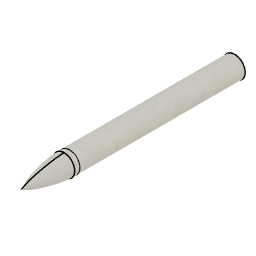
Rocket- Main Body with nosecone_ (Autodesk Fusion 360 design; units mm, degrees)
Autodesk Fusion 360 part; units mm, degrees
sketch "Rocket Nose" plane through (0, 0, 0) normal (1, 0, 0) x (0, 1, 0)
  spline S0 degree 5 poles (152.4, 0) (151.241, 0.6822) (148.9185, 2.0223) (145.4215, 3.9595) (140.7321, 6.3961) (134.8257, 9.1975) (128.8755, 11.7569) (122.883, 14.0821) (116.8517, 16.1887) (110.7874, 18.1036) (104.6973, 19.8612) (98.589, 21.4976) (92.4695, 23.0466) (86.3443, 24.5345) (80.2158, 25.9747) (74.0842, 27.3699) (67.9484, 28.7154) (61.8067, 30.0021) (55.6572, 31.2194) (49.4994, 32.3582) (43.3333, 33.4116) (37.1596, 34.3742) (30.9793, 35.2422) (24.7932, 36.0132) (18.602, 36.6866) (12.4061, 37.2623) (7.4458, 37.6454) (3.7237, 37.8895) (1.2414, 38.033) (0, 38.1) knots 0 0 0 0 0 0 0.04 0.08 0.12 0.16 0.2 0.24 0.28 0.32 0.36 0.4 0.44 0.48 0.52 0.56 0.6 0.64 0.68 0.72 0.76 0.8 0.84 0.88 0.92 0.96 1 1 1 1 1 1
  line L0 (152.4, 0) -> (-19.0521, 0)
  line L1 (-19.0521, 0) -> (-19.0521, 36.8301)
  line L2 (-19.0521, 36.8301) -> (0, 36.8301)
  line L3 (0, 36.8301) -> (0, 38.1)
  line L4 (0, 16) -> (-19.05, 16) construction
  line L5 (0, 38.1) -> (-19.4564, 38.1) construction
  line L6 (-9.7282, 38.1) -> (-9.7282, 36.83) construction
  point P0 (121.92, 14.3763)
  point P1 (91.44, 23.2856)
  point P2 (60.96, 30.1561)
  point P3 (30.48, 35.2836)
  dimension "d13" = 19.05
  dimension "d20" = 1.27
  constraint perpendicular L1 L4
  constraint perpendicular L3 L5
  constraint midpoint L5 L6.start
  constraint perpendicular L2 L6
  measures "d13" distance of L4.start L4.end
  measures "d20" distance of L6.start L6.end
revolve "Revolve1" add sketch "Rocket Nose" angle 360 about axis through (0, 152.4, 0) along (0, -1, 0) makes body 1
sketch "Structure Cylinder" plane through (0, 0, 0) normal (0, 1, 0) x (1, 0, 0)
  circle A0 centre (0, 0) radius 38.1
  circle A1 centre (0, 0) radius 36.9094
  dimension "d2" = 76.2
  dimension "d6" = -1.1906
  constraint coincident A0.centre A1.centre
  measures "d2" diameter of A0
move_body "Move1" bodies 1 to x (1, 0, 0) y (0, 1, 0) z (0, 0, 1) at (-175.7241, -67.6703, 17.5352)
extrude "Extrude2" add sketch "Structure Cylinder" along normal blind 609.6 separate body makes body 2
move_body "Move2" bodies 1 to x (-1, 0, 0) y (0, -1, 0) z (0, 0, 1) at (0, 0, 0)
move_body "Move3" bodies 1 to x (1, 0, 0) y (0, 1, 0) z (0, 0, 1) at (-164.1367, -284.7307, -9.893)
move_body "Move4" bodies 1 to x (1, 0, 0) y (0, 1, 0) z (0, 0, 1) at (-11.5874, 198.0083, -7.6422)
move_body "Move5" bodies 1 to x (1, 0, 0) y (0, 1, 0) z (0, 0, 1) at (0, 50.8, 0)
sketch "Nose and Structure" plane through (0, 0, 0) normal (0, 0, 1) x (1, 0, 0)
  line L0 (38.1, 609.6) -> (-38.1, 609.6)
  line L1 (38.1, 0) -> (-38.1, 0)
  line L2 (38.1, 0) -> (38.1, 609.6)
  line L3 (-38.1, 0) -> (-38.1, 609.6)
  line L4 (-36.8301, 50.8) -> (36.8301, 50.8)
  line L5 (-38.1, 31.7479) -> (-36.8301, 31.7479)
  line L6 (36.8301, 31.7479) -> (38.1, 31.7479)
  line L7 (-36.8301, 50.8) -> (-36.8301, 31.7479)
  line L8 (36.8301, 50.8) -> (36.8301, 31.7479)
  spline S0 degree 3 poles (0, -120.6521) (-5.685, -110.9936) (-10.3314, -101.1446) (-17.7236, -81.1062) (-20.4978, -70.9235) (-25.5647, -50.5168) (-27.8995, -40.2997) (-32.07, -19.814) (-33.8523, -9.5352) (-36.5836, 11.0753) (-37.5419, 21.4031) (-38.1, 31.7479) knots 0 0 0 0 0.2 0.2 0.4 0.4 0.6 0.6 0.8 0.8 1 1 1 1
  spline S1 degree 3 poles (0, -120.6521) (5.685, -110.9936) (10.3314, -101.1446) (17.7236, -81.1062) (20.4978, -70.9235) (25.5647, -50.5168) (27.8995, -40.2997) (32.07, -19.814) (33.8523, -9.5352) (36.5836, 11.0753) (37.5419, 21.4031) (38.1, 31.7479) knots 0 0 0 0 0.2 0.2 0.4 0.4 0.6 0.6 0.8 0.8 1 1 1 1
move_body "Move6" bodies 1 to x (1, 0, 0) y (0, 1, 0) z (0, 0, 1) at (0, -40, 0)
move_body "Move7" bodies 1 to x (1, 0, 0) y (0, 1, 0) z (0, 0, 1) at (0, 8.3, 0)
named bodies: "Nose Cone (Zero Drag)", "Rocket Structure"
